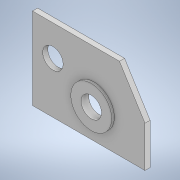
# Autodesk Inventor part: Assignment 3.2 - Guide Plate
Saved by Autodesk Inventor 2022 (Build 260153000, 153)
## iProperties
Created: 2021-05-23
Part Number: Assignment 3.2 - Guide Plate
Material: Generic
Document SubType Name: Modeling
Designer: Aaron
Density: 1 g/cm^3
Appearance: Default
Author: Aaron
Autodesk Inventor part; units mm, degrees
ref_plane "YZ Plane" through (0, 0, 0) normal (1, 0, 0) x (0, 1, 0)
ref_plane "XZ Plane" through (0, 0, 0) normal (0, 1, 0) x (-1, 0, 0)
ref_plane "XY Plane" through (0, 0, 0) normal (0, 0, 1) x (1, 0, 0)
sketch "Sketch1" plane through (0, 0, 0) normal (0, 0, 1) x (1, 0, 0)
  line L0 (0, 0) -> (0, 101.6)
  line L1 (0, 101.6) -> (107.95, 101.6)
  circle A0 centre (76.2, 38.1) radius 12.7
  circle A1 centre (76.2, 38.1) radius 25.4
  circle A2 centre (25.4, 63.5) radius 12.7
  line L2 (0, 0) -> (139.7, 0)
  line L3 (139.7, 0) -> (139.7, 50.8)
  line L4 (139.7, 50.8) -> (107.95, 101.6)
  dimension "d0" = 101.6
  dimension "d1" = 107.95
  dimension "d4" = 25.4
  dimension "d5" = 50.8
  dimension "d8" = 25.4
  dimension "d9" = 139.7
  dimension "d11" = 50.8
  constraints: 10 end point, 3 centre point, 2 vertical, 1 coincident, 1 horizontal, 1 perpendicular
  measures "d0" distance of L0.start L0.end
  measures "d1" distance of L0.end L1.end
  measures "d4" diameter of A0
  measures "d5" diameter of A1
  measures "d8" diameter of A2
  measures "d9" distance of L0.start L2.end
  measures "d11" distance of L2.end L3.end
extrude "Extrusion1" add sketch "Sketch1" along normal blind 6.35 contours L0 L1 L4 L3 L2
sketch "Sketch2" plane through (0, 0, 6.35) normal (0, 0, 1) x (1, 0, 0)
  circle A0 centre (76.2, 38.1) radius 12.7
  circle A1 centre (76.2, 38.1) radius 25.4
  point P0 (0, 0)
  dimension "d16" = 25.4
  constraints: 2 centre point, 1 coincident
  measures "d16" diameter of A0
extrude "Extrusion2" add sketch "Sketch2" along normal blind 3.175 and the other way blind 6.35
body "Solid1"
